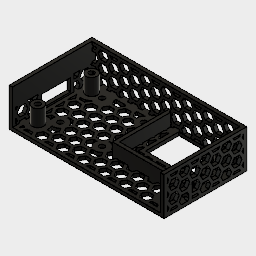
Enclosure Bottom (Autodesk Fusion 360 design; units mm, degrees)
Autodesk Fusion 360 part; units mm, degrees
(part 1 of 2)
sketch "Base and Side Wall" plane through (0, 0, 0) normal (0, 1, 0) x (1, 0, 0)
  line L0 (0, 0) -> (88.9, 0)
  line L1 (88.9, 0) -> (88.9, -47.6)
  line L2 (88.9, -47.6) -> (0, -47.6)
  line L3 (0, -47.6) -> (0, 0)
  line L4 (0, 0) -> (0, -2)
  line L5 (2, -2) -> (86.9, -2)
  line L6 (86.9, -2) -> (86.9, -47.6)
  line L7 (2, -47.6) -> (2, -2)
  dimension "d1" = 88.9
  dimension "d2" = 47.6
  dimension "d3" = 2
  dimension "d100" = 2
  measures "d1" distance of L0.start L0.end
  measures "d2" distance of L0.start L2.end
  measures "d3" distance of L0.start L4.end
extrude "Extrude1" add sketch "Base and Side Wall" along normal blind 2 contours L2 L5 L6 L7 makes body 1
extrude "Extrude2" add sketch "Base and Side Wall" along normal blind 22 separate body contours L0 L1 L2 L3 L4 L5 L6 L7 makes body 2
sketch "Board Construction Lines" plane through (0, 0, 0) normal (0, 1, 0) x (1, 0, 0)
  line L0 (4.75, -3.4956) -> (85.4, -3.5) construction
  line L1 (85.4, -3.5) -> (85.3525, -46.1425) construction
  line L2 (85.3525, -46.1425) -> (4.7511, -46.1014) construction
  line L3 (4.7511, -46.1014) -> (4.75, -3.4956) construction
  line L4 (4.75, -3.4956) -> (7.15, -3.5001) construction
  line L5 (7.15, -3.5001) -> (7.1569, -7.3501) construction
  line L6 (7.1569, -7.3501) -> (4.7569, -7.3456) construction
  line L7 (4.7569, -7.3456) -> (4.75, -3.4956) construction
  line L8 (85.4, -3.5) -> (82.15, -3.5001) construction
  line L9 (82.15, -3.5001) -> (82.1501, -7.3501) construction
  line L10 (82.1501, -7.3501) -> (85.4001, -7.35) construction
  line L11 (85.4001, -7.35) -> (85.4, -3.5) construction
  line L12 (4.7511, -46.1014) -> (7.1511, -46.1012) construction
  line L13 (7.1511, -46.1012) -> (7.1569, -38.2512) construction
  line L14 (7.1569, -38.2512) -> (4.7569, -38.2514) construction
  line L15 (4.7569, -38.2514) -> (4.7511, -46.1014) construction
  line L16 (85.3525, -46.1425) -> (82.1027, -46.1011) construction
  line L17 (82.1027, -46.1011) -> (82.1501, -38.2512) construction
  line L18 (82.1501, -38.2512) -> (85.3999, -38.2926) construction
  line L19 (85.3999, -38.2926) -> (85.3525, -46.1425) construction
  line L20 (7.1569, -7.3501) -> (82.1501, -7.3501) construction
  line L21 (82.1501, -7.3501) -> (82.1501, -38.2512) construction
  line L22 (82.1501, -38.2512) -> (7.1569, -38.2512) construction
  line L23 (7.1569, -38.2512) -> (7.1569, -7.3501) construction
  dimension "d18" = 80.65
  dimension "d20" = 2.4
  dimension "d21" = 3.25
  dimension "d22" = 3.85
  dimension "d23" = 7.85
  measures "d18" distance of L0.start L0.end
  measures "d20" distance of L0.start L4.end
  measures "d21" distance of L0.end L8.end
  measures "d22" distance of L0.end L10.end
  measures "d23" distance of L2.end L14.end
sketch "Standoffs" plane through (0, 2, 0) normal (0, 1, 0) x (-1, 0, 0)
  line L0 (-2, 47.6) -> (-86.9, 47.6)
  line L1 (-86.9, 47.6) -> (-86.9, 2)
  line L2 (-86.9, 2) -> (-2, 2)
  line L3 (-2, 2) -> (-2, 47.6)
  circle A0 centre (-7.1569, 7.3501) radius 1.5
  circle A1 centre (-7.147, 7.3545) radius 3.25
  circle A2 centre (-7.147, 7.3545) radius 1.5
  circle A3 centre (-82.1501, 7.3501) radius 1.5
  circle A4 centre (-82.1501, 7.3501) radius 3.25
  circle A5 centre (-82.1501, 38.2512) radius 1.5
  circle A6 centre (-82.1501, 38.2512) radius 3.25
  circle A7 centre (-7.1569, 38.2512) radius 1.5
  circle A8 centre (-7.1569, 38.2512) radius 3.25
  point P0 (-7.1569, 7.3501)
  point P1 (-82.1501, 7.3501)
  point P2 (-82.1501, 38.2512)
  point P3 (-7.1569, 38.2512)
  dimension "d29" = 3
  dimension "d31" = 3
  dimension "d32" = 6.5
  dimension "d33" = 3
  dimension "d34" = 6.5
  dimension "d37" = 3
  dimension "d38" = 6.5
  dimension "d41" = 3
  dimension "d42" = 6.5
  measures "d29" diameter of A0
  measures "d31" diameter of A2
  measures "d32" diameter of A1
  measures "d33" diameter of A3
  measures "d34" diameter of A4
  measures "d37" diameter of A5
  measures "d38" diameter of A6
  measures "d41" diameter of A7
  measures "d42" diameter of A8
extrude "Extrude3" add sketch "Standoffs" along normal blind 9.5 contours A1 | A4 | A6 bodies 1
sketch "Nut Holes" plane through (0, 0, 0) normal (0, 1, 0) x (1, 0, 0)
  line L0 (9.4069, -38.2546) -> (8.2848, -36.3043)
  line L1 (8.2848, -36.3043) -> (6.0348, -36.301)
  line L2 (6.0348, -36.301) -> (4.9069, -38.2478)
  line L3 (4.9069, -38.2478) -> (6.029, -40.1981)
  line L4 (6.029, -40.1981) -> (8.279, -40.2014)
  line L5 (8.279, -40.2014) -> (9.4069, -38.2546)
  line L6 (79.9001, -38.2512) -> (81.0251, -40.1998)
  line L7 (81.0251, -40.1998) -> (83.2751, -40.1998)
  line L8 (83.2751, -40.1998) -> (84.4001, -38.2512)
  line L9 (84.4001, -38.2512) -> (83.2751, -36.3026)
  line L10 (83.2751, -36.3026) -> (81.0251, -36.3026)
  line L11 (81.0251, -36.3026) -> (79.9001, -38.2512)
  line L12 (79.9001, -7.3501) -> (81.0251, -9.2987)
  line L13 (81.0251, -9.2987) -> (83.2751, -9.2987)
  line L14 (83.2751, -9.2987) -> (84.4001, -7.3501)
  line L15 (84.4001, -7.3501) -> (83.2751, -5.4016)
  line L16 (83.2751, -5.4016) -> (81.0251, -5.4016)
  line L17 (81.0251, -5.4016) -> (79.9001, -7.3501)
  line L18 (9.397, -7.3528) -> (8.2705, -5.4051)
  line L19 (8.2705, -5.4051) -> (6.0205, -5.4069)
  line L20 (6.0205, -5.4069) -> (4.897, -7.3563)
  line L21 (4.897, -7.3563) -> (6.0236, -9.304)
  line L22 (6.0236, -9.304) -> (8.2736, -9.3022)
  line L23 (8.2736, -9.3022) -> (9.397, -7.3528)
  point P0 (7.1569, -38.2512)
  point P1 (82.1501, -38.2512)
  point P2 (82.1501, -7.3501)
  point P3 (7.147, -7.3545)
  dimension "d205" = 4.5
  dimension "d206" = 4.5
  dimension "d207" = 4.5
  dimension "d208" = 4.5
  measures "d205" distance of L0.start L2.end
  measures "d206" distance of L6.start L8.end
  measures "d207" distance of L18.start L20.end
  measures "d208" distance of L12.start L14.end
extrude "Extrude4" add sketch "Standoffs" along normal blind 9.5 contours A8 bodies 1
extrude "Extrude5" cut sketch "Nut Holes" along normal blind 6 bodies 1
sketch "USB Port" plane through (0, 0, 0) normal (1, 0, 0) x (0, 0, -1)
  line L0 (-30.93, 3) -> (-14.33, 3)
  line L1 (-14.33, 3) -> (-14.33, 10)
  line L2 (-14.33, 10) -> (-30.93, 10)
  line L3 (-30.93, 10) -> (-30.93, 3)
  point P0 (-20.63, 6.5)
  point P1 (-20.63, 6.5)
  dimension "d49" = 16.6
  dimension "d50" = 7
  measures "d49" distance of L1.end L2.end
  measures "d50" distance of L0.end L1.end
extrude "Extrude6" cut sketch "USB Port" along normal blind 2 bodies 2
sketch "Bottom Honeycomb" plane through (0, 0, 0) normal (0, 1, 0) x (1, 0, 0)
  line L0 (77.1501, -5.9981) -> (12.1569, -5.9981) construction
  line L1 (12.1569, -5.9981) -> (12.1569, -45.6006) construction
  line L2 (12.1569, -45.6006) -> (77.1501, -45.6006) construction
  line L3 (77.1501, -45.6006) -> (77.1501, -5.9981) construction
  line L4 (47.6535, -25.7993) -> (46.1535, -23.2013)
  line L5 (46.1535, -23.2013) -> (43.1535, -23.2013)
  line L6 (43.1535, -23.2013) -> (41.6535, -25.7993)
  line L7 (41.6535, -25.7993) -> (43.1535, -28.3974)
  line L8 (43.1535, -28.3974) -> (46.1535, -28.3974)
  line L9 (46.1535, -28.3974) -> (47.6535, -25.7993)
  line L10 (41.6535, -29.2993) -> (40.1535, -26.7013)
  line L11 (40.1535, -26.7013) -> (37.1535, -26.7013)
  line L12 (37.1535, -26.7013) -> (35.6535, -29.2993)
  line L13 (35.6535, -29.2993) -> (37.1535, -31.8974)
  line L14 (37.1535, -31.8974) -> (40.1535, -31.8974)
  line L15 (40.1535, -31.8974) -> (41.6535, -29.2993)
  line L16 (35.6535, -25.7993) -> (34.1535, -23.2013)
  line L17 (34.1535, -23.2013) -> (31.1535, -23.2013)
  line L18 (31.1535, -23.2013) -> (29.6535, -25.7993)
  line L19 (29.6535, -25.7993) -> (31.1535, -28.3974)
  line L20 (31.1535, -28.3974) -> (34.1535, -28.3974)
  line L21 (34.1535, -28.3974) -> (35.6535, -25.7993)
  line L22 (22.1535, -23.2013) -> (19.1535, -23.2013)
  line L23 (19.1535, -23.2013) -> (17.6535, -25.7993)
  line L24 (17.6535, -25.7993) -> (19.1535, -28.3974)
  line L25 (19.1535, -28.3974) -> (22.1535, -28.3974)
  line L26 (22.1535, -28.3974) -> (23.6535, -25.7993)
  line L27 (23.6535, -25.7993) -> (22.1535, -23.2013)
  line L28 (11.6535, -25.7993) -> (10.1535, -23.2013)
  line L29 (10.1535, -23.2013) -> (7.1535, -23.2013)
  line L30 (7.1535, -23.2013) -> (5.6535, -25.7993)
  line L31 (5.6535, -25.7993) -> (7.1535, -28.3974)
  line L32 (7.1535, -28.3974) -> (10.1535, -28.3974)
  line L33 (10.1535, -28.3974) -> (11.6535, -25.7993)
  line L34 (59.6535, -25.7993) -> (58.1535, -23.2013)
  line L35 (58.1535, -23.2013) -> (55.1535, -23.2013)
  line L36 (55.1535, -23.2013) -> (53.6535, -25.7993)
  line L37 (53.6535, -25.7993) -> (55.1535, -28.3974)
  line L38 (55.1535, -28.3974) -> (58.1535, -28.3974)
  line L39 (58.1535, -28.3974) -> (59.6535, -25.7993)
  line L40 (71.6535, -25.7993) -> (70.1535, -23.2013)
  line L41 (70.1535, -23.2013) -> (67.1535, -23.2013)
  line L42 (67.1535, -23.2013) -> (65.6535, -25.7993)
  line L43 (65.6535, -25.7993) -> (67.1535, -28.3974)
  line L44 (67.1535, -28.3974) -> (70.1535, -28.3974)
  line L45 (70.1535, -28.3974) -> (71.6535, -25.7993)
  line L46 (83.6535, -25.7993) -> (82.1535, -23.2013)
  line L47 (82.1535, -23.2013) -> (79.1535, -23.2013)
  line L48 (79.1535, -23.2013) -> (77.6535, -25.7993)
  line L49 (77.6535, -25.7993) -> (79.1535, -28.3974)
  line L50 (79.1535, -28.3974) -> (82.1535, -28.3974)
  line L51 (82.1535, -28.3974) -> (83.6535, -25.7993)
  line L52 (29.6535, -29.2993) -> (28.1535, -26.7013)
  line L53 (28.1535, -26.7013) -> (25.1535, -26.7013)
  line L54 (25.1535, -26.7013) -> (23.6535, -29.2993)
  line L55 (23.6535, -29.2993) -> (25.1535, -31.8974)
  line L56 (25.1535, -31.8974) -> (28.1535, -31.8974)
  line L57 (28.1535, -31.8974) -> (29.6535, -29.2993)
  line L58 (16.1535, -26.7013) -> (13.1535, -26.7013)
  line L59 (13.1535, -26.7013) -> (11.6535, -29.2993)
  line L60 (11.6535, -29.2993) -> (13.1535, -31.8974)
  line L61 (13.1535, -31.8974) -> (16.1535, -31.8974)
  line L62 (16.1535, -31.8974) -> (17.6535, -29.2993)
  line L63 (17.6535, -29.2993) -> (16.1535, -26.7013)
  line L64 (53.6535, -29.2993) -> (52.1535, -26.7013)
  line L65 (52.1535, -26.7013) -> (49.1535, -26.7013)
  line L66 (49.1535, -26.7013) -> (47.6535, -29.2993)
  line L67 (47.6535, -29.2993) -> (49.1535, -31.8974)
  line L68 (49.1535, -31.8974) -> (52.1535, -31.8974)
  line L69 (52.1535, -31.8974) -> (53.6535, -29.2993)
  line L70 (65.6535, -29.2993) -> (64.1535, -26.7013)
  line L71 (64.1535, -26.7013) -> (61.1535, -26.7013)
  line L72 (61.1535, -26.7013) -> (59.6535, -29.2993)
  line L73 (59.6535, -29.2993) -> (61.1535, -31.8974)
  line L74 (61.1535, -31.8974) -> (64.1535, -31.8974)
  line L75 (64.1535, -31.8974) -> (65.6535, -29.2993)
  line L76 (76.1535, -26.7013) -> (73.1535, -26.7013)
  line L77 (73.1535, -26.7013) -> (71.6535, -29.2993)
  line L78 (71.6535, -29.2993) -> (73.1535, -31.8974)
  line L79 (73.1535, -31.8974) -> (76.1535, -31.8974)
  line L80 (76.1535, -31.8974) -> (77.6535, -29.2993)
  line L81 (77.6535, -29.2993) -> (76.1535, -26.7013)
  line L82 (17.6535, -22.2993) -> (16.1535, -19.7013)
  line L83 (16.1535, -19.7013) -> (13.1535, -19.7013)
  line L84 (13.1535, -19.7013) -> (11.6535, -22.2993)
  line L85 (11.6535, -22.2993) -> (13.1535, -24.8974)
  line L86 (13.1535, -24.8974) -> (16.1535, -24.8974)
  line L87 (16.1535, -24.8974) -> (17.6535, -22.2993)
  line L88 (29.6535, -22.2993) -> (28.1535, -19.7013)
  line L89 (28.1535, -19.7013) -> (25.1535, -19.7013)
  line L90 (25.1535, -19.7013) -> (23.6535, -22.2993)
  line L91 (23.6535, -22.2993) -> (25.1535, -24.8974)
  line L92 (28.1535, -24.8974) -> (29.6535, -22.2993)
  line L93 (25.1535, -24.8974) -> (28.1535, -24.8974)
  line L94 (41.6535, -22.2993) -> (40.1535, -19.7013)
  line L95 (40.1535, -19.7013) -> (37.1535, -19.7013)
  line L96 (37.1535, -19.7013) -> (35.6535, -22.2993)
  line L97 (35.6535, -22.2993) -> (37.1535, -24.8974)
  line L98 (40.1535, -24.8974) -> (41.6535, -22.2993)
  line L99 (37.1535, -24.8974) -> (40.1535, -24.8974)
  line L100 (53.6535, -22.2993) -> (52.1535, -19.7013)
  line L101 (52.1535, -19.7013) -> (49.1535, -19.7013)
  line L102 (49.1535, -19.7013) -> (47.6535, -22.2993)
  line L103 (47.6535, -22.2993) -> (49.1535, -24.8974)
  line L104 (52.1535, -24.8974) -> (53.6535, -22.2993)
  line L105 (49.1535, -24.8974) -> (52.1535, -24.8974)
  line L106 (65.6535, -22.2993) -> (64.1535, -19.7013)
  line L107 (64.1535, -19.7013) -> (61.1535, -19.7013)
  line L108 (61.1535, -19.7013) -> (59.6535, -22.2993)
  line L109 (59.6535, -22.2993) -> (61.1535, -24.8974)
  line L110 (64.1535, -24.8974) -> (65.6535, -22.2993)
  line L111 (61.1535, -24.8974) -> (64.1535, -24.8974)
  line L112 (77.6535, -22.2993) -> (76.1535, -19.7013)
  line L113 (76.1535, -19.7013) -> (73.1535, -19.7013)
  line L114 (73.1535, -19.7013) -> (71.6535, -22.2993)
  line L115 (71.6535, -22.2993) -> (73.1535, -24.8974)
  line L116 (76.1535, -24.8974) -> (77.6535, -22.2993)
  line L117 (73.1535, -24.8974) -> (76.1535, -24.8974)
  line L118 (11.6535, -18.7993) -> (10.1535, -16.2013)
  line L119 (10.1535, -16.2013) -> (7.1535, -16.2013)
  line L120 (7.1535, -16.2013) -> (5.6535, -18.7993)
  line L121 (5.6535, -18.7993) -> (7.1535, -21.3974)
  line L122 (7.1535, -21.3974) -> (10.1535, -21.3974)
  line L123 (10.1535, -21.3974) -> (11.6535, -18.7993)
  line L124 (23.6535, -18.7993) -> (22.1535, -16.2013)
  line L125 (22.1535, -16.2013) -> (19.1535, -16.2013)
  line L126 (19.1535, -16.2013) -> (17.6535, -18.7993)
  line L127 (17.6535, -18.7993) -> (19.1535, -21.3974)
  line L128 (22.1535, -21.3974) -> (23.6535, -18.7993)
  line L129 (19.1535, -21.3974) -> (22.1535, -21.3974)
  line L130 (35.6535, -18.7993) -> (34.1535, -16.2013)
  line L131 (34.1535, -16.2013) -> (31.1535, -16.2013)
  line L132 (31.1535, -16.2013) -> (29.6535, -18.7993)
  line L133 (29.6535, -18.7993) -> (31.1535, -21.3974)
  line L134 (34.1535, -21.3974) -> (35.6535, -18.7993)
  line L135 (31.1535, -21.3974) -> (34.1535, -21.3974)
  line L136 (47.6535, -18.7993) -> (46.1535, -16.2013)
  line L137 (46.1535, -16.2013) -> (43.1535, -16.2013)
  line L138 (43.1535, -16.2013) -> (41.6535, -18.7993)
  line L139 (41.6535, -18.7993) -> (43.1535, -21.3974)
  line L140 (46.1535, -21.3974) -> (47.6535, -18.7993)
  line L141 (43.1535, -21.3974) -> (46.1535, -21.3974)
  line L142 (59.6535, -18.7993) -> (58.1535, -16.2013)
  line L143 (58.1535, -16.2013) -> (55.1535, -16.2013)
  line L144 (55.1535, -16.2013) -> (53.6535, -18.7993)
  line L145 (53.6535, -18.7993) -> (55.1535, -21.3974)
  line L146 (58.1535, -21.3974) -> (59.6535, -18.7993)
  line L147 (55.1535, -21.3974) -> (58.1535, -21.3974)
  line L148 (71.6535, -18.7993) -> (70.1535, -16.2013)
  line L149 (70.1535, -16.2013) -> (67.1535, -16.2013)
  line L150 (67.1535, -16.2013) -> (65.6535, -18.7993)
  line L151 (65.6535, -18.7993) -> (67.1535, -21.3974)
  line L152 (70.1535, -21.3974) -> (71.6535, -18.7993)
  line L153 (67.1535, -21.3974) -> (70.1535, -21.3974)
  line L154 (83.6535, -18.7993) -> (82.1535, -16.2013)
  line L155 (82.1535, -16.2013) -> (79.1535, -16.2013)
  line L156 (79.1535, -16.2013) -> (77.6535, -18.7993)
  line L157 (77.6535, -18.7993) -> (79.1535, -21.3974)
  line L158 (82.1535, -21.3974) -> (83.6535, -18.7993)
  line L159 (79.1535, -21.3974) -> (82.1535, -21.3974)
  line L160 (23.6535, -11.7993) -> (22.1535, -9.2013)
  line L161 (22.1535, -9.2013) -> (19.1535, -9.2013)
  line L162 (19.1535, -9.2013) -> (17.6535, -11.7993)
  line L163 (17.6535, -11.7993) -> (19.1535, -14.3974)
  line L164 (22.1535, -14.3974) -> (23.6535, -11.7993)
  line L165 (19.1535, -14.3974) -> (22.1535, -14.3974)
  line L166 (35.6535, -11.7993) -> (34.1535, -9.2013)
  line L167 (34.1535, -9.2013) -> (31.1535, -9.2013)
  line L168 (31.1535, -9.2013) -> (29.6535, -11.7993)
  line L169 (29.6535, -11.7993) -> (31.1535, -14.3974)
  line L170 (34.1535, -14.3974) -> (35.6535, -11.7993)
  line L171 (31.1535, -14.3974) -> (34.1535, -14.3974)
  line L172 (47.6535, -11.7993) -> (46.1535, -9.2013)
  line L173 (46.1535, -9.2013) -> (43.1535, -9.2013)
  line L174 (43.1535, -9.2013) -> (41.6535, -11.7993)
  line L175 (41.6535, -11.7993) -> (43.1535, -14.3974)
  line L176 (46.1535, -14.3974) -> (47.6535, -11.7993)
  line L177 (43.1535, -14.3974) -> (46.1535, -14.3974)
  line L178 (59.6535, -11.7993) -> (58.1535, -9.2013)
  line L179 (58.1535, -9.2013) -> (55.1535, -9.2013)
  line L180 (55.1535, -9.2013) -> (53.6535, -11.7993)
  line L181 (53.6535, -11.7993) -> (55.1535, -14.3974)
  line L182 (58.1535, -14.3974) -> (59.6535, -11.7993)
  line L183 (55.1535, -14.3974) -> (58.1535, -14.3974)
  line L184 (71.6535, -11.7993) -> (70.1535, -9.2013)
  line L185 (70.1535, -9.2013) -> (67.1535, -9.2013)
  line L186 (67.1535, -9.2013) -> (65.6535, -11.7993)
  line L187 (65.6535, -11.7993) -> (67.1535, -14.3974)
  line L188 (70.1535, -14.3974) -> (71.6535, -11.7993)
  line L189 (67.1535, -14.3974) -> (70.1535, -14.3974)
  line L190 (17.6535, -15.2993) -> (16.1535, -12.7013)
  line L191 (16.1535, -12.7013) -> (13.1535, -12.7013)
  line L192 (13.1535, -12.7013) -> (11.6535, -15.2993)
  line L193 (11.6535, -15.2993) -> (13.1535, -17.8974)
  line L194 (13.1535, -17.8974) -> (16.1535, -17.8974)
  line L195 (16.1535, -17.8974) -> (17.6535, -15.2993)
  line L196 (29.6535, -15.2993) -> (28.1535, -12.7013)
  line L197 (28.1535, -12.7013) -> (25.1535, -12.7013)
  line L198 (25.1535, -12.7013) -> (23.6535, -15.2993)
  line L199 (23.6535, -15.2993) -> (25.1535, -17.8974)
  line L200 (28.1535, -17.8974) -> (29.6535, -15.2993)
  line L201 (25.1535, -17.8974) -> (28.1535, -17.8974)
  line L202 (41.6535, -15.2993) -> (40.1535, -12.7013)
  line L203 (40.1535, -12.7013) -> (37.1535, -12.7013)
  line L204 (37.1535, -12.7013) -> (35.6535, -15.2993)
  line L205 (35.6535, -15.2993) -> (37.1535, -17.8974)
  line L206 (40.1535, -17.8974) -> (41.6535, -15.2993)
  line L207 (37.1535, -17.8974) -> (40.1535, -17.8974)
  line L208 (53.6535, -15.2993) -> (52.1535, -12.7013)
  line L209 (52.1535, -12.7013) -> (49.1535, -12.7013)
  line L210 (49.1535, -12.7013) -> (47.6535, -15.2993)
  line L211 (47.6535, -15.2993) -> (49.1535, -17.8974)
  line L212 (52.1535, -17.8974) -> (53.6535, -15.2993)
  line L213 (49.1535, -17.8974) -> (52.1535, -17.8974)
  line L214 (65.6535, -15.2993) -> (64.1535, -12.7013)
  line L215 (64.1535, -12.7013) -> (61.1535, -12.7013)
  line L216 (61.1535, -12.7013) -> (59.6535, -15.2993)
  line L217 (59.6535, -15.2993) -> (61.1535, -17.8974)
  line L218 (64.1535, -17.8974) -> (65.6535, -15.2993)
  line L219 (61.1535, -17.8974) -> (64.1535, -17.8974)
  line L220 (77.6535, -15.2993) -> (76.1535, -12.7013)
  line L221 (76.1535, -12.7013) -> (73.1535, -12.7013)
  line L222 (73.1535, -12.7013) -> (71.6535, -15.2993)
  line L223 (71.6535, -15.2993) -> (73.1535, -17.8974)
  line L224 (76.1535, -17.8974) -> (77.6535, -15.2993)
  line L225 (73.1535, -17.8974) -> (76.1535, -17.8974)
  line L226 (23.6535, -32.7993) -> (22.1535, -30.2013)
  line L227 (22.1535, -30.2013) -> (19.1535, -30.2013)
  line L228 (19.1535, -30.2013) -> (17.6535, -32.7993)
  line L229 (17.6535, -32.7993) -> (19.1535, -35.3974)
  line L230 (22.1535, -35.3974) -> (23.6535, -32.7993)
  line L231 (19.1535, -35.3974) -> (22.1535, -35.3974)
  line L232 (35.6535, -32.7993) -> (34.1535, -30.2013)
  line L233 (34.1535, -30.2013) -> (31.1535, -30.2013)
  line L234 (31.1535, -30.2013) -> (29.6535, -32.7993)
  line L235 (29.6535, -32.7993) -> (31.1535, -35.3974)
  line L236 (34.1535, -35.3974) -> (35.6535, -32.7993)
  line L237 (31.1535, -35.3974) -> (34.1535, -35.3974)
  line L238 (47.6535, -32.7993) -> (46.1535, -30.2013)
  line L239 (46.1535, -30.2013) -> (43.1535, -30.2013)
  line L240 (43.1535, -30.2013) -> (41.6535, -32.7993)
  line L241 (41.6535, -32.7993) -> (43.1535, -35.3974)
  line L242 (46.1535, -35.3974) -> (47.6535, -32.7993)
  line L243 (43.1535, -35.3974) -> (46.1535, -35.3974)
  line L244 (59.6535, -32.7993) -> (58.1535, -30.2013)
  line L245 (58.1535, -30.2013) -> (55.1535, -30.2013)
  line L246 (55.1535, -30.2013) -> (53.6535, -32.7993)
  line L247 (53.6535, -32.7993) -> (55.1535, -35.3974)
  line L248 (58.1535, -35.3974) -> (59.6535, -32.7993)
  line L249 (55.1535, -35.3974) -> (58.1535, -35.3974)
  line L250 (71.6535, -32.7993) -> (70.1535, -30.2013)
  line L251 (70.1535, -30.2013) -> (67.1535, -30.2013)
  line L252 (67.1535, -30.2013) -> (65.6535, -32.7993)
  line L253 (65.6535, -32.7993) -> (67.1535, -35.3974)
  line L254 (70.1535, -35.3974) -> (71.6535, -32.7993)
  line L255 (67.1535, -35.3974) -> (70.1535, -35.3974)
  line L256 (17.6535, -36.2993) -> (16.1535, -33.7013)
  line L257 (16.1535, -33.7013) -> (13.1535, -33.7013)
  line L258 (13.1535, -33.7013) -> (11.6535, -36.2993)
  line L259 (11.6535, -36.2993) -> (13.1535, -38.8974)
  line L260 (13.1535, -38.8974) -> (16.1535, -38.8974)
  line L261 (16.1535, -38.8974) -> (17.6535, -36.2993)
  line L262 (29.6535, -36.2993) -> (28.1535, -33.7013)
  line L263 (28.1535, -33.7013) -> (25.1535, -33.7013)
  line L264 (25.1535, -33.7013) -> (23.6535, -36.2993)
  line L265 (23.6535, -36.2993) -> (25.1535, -38.8974)
  line L266 (28.1535, -38.8974) -> (29.6535, -36.2993)
  line L267 (25.1535, -38.8974) -> (28.1535, -38.8974)
  line L268 (41.6535, -36.2993) -> (40.1535, -33.7013)
  line L269 (40.1535, -33.7013) -> (37.1535, -33.7013)
  line L270 (37.1535, -33.7013) -> (35.6535, -36.2993)
  line L271 (35.6535, -36.2993) -> (37.1535, -38.8974)
  line L272 (40.1535, -38.8974) -> (41.6535, -36.2993)
  line L273 (37.1535, -38.8974) -> (40.1535, -38.8974)
  line L274 (53.6535, -36.2993) -> (52.1535, -33.7013)
  line L275 (52.1535, -33.7013) -> (49.1535, -33.7013)
  line L276 (49.1535, -33.7013) -> (47.6535, -36.2993)
  line L277 (47.6535, -36.2993) -> (49.1535, -38.8974)
  line L278 (52.1535, -38.8974) -> (53.6535, -36.2993)
  line L279 (49.1535, -38.8974) -> (52.1535, -38.8974)
  line L280 (65.6535, -36.2993) -> (64.1535, -33.7013)
  line L281 (64.1535, -33.7013) -> (61.1535, -33.7013)
  line L282 (61.1535, -33.7013) -> (59.6535, -36.2993)
  line L283 (59.6535, -36.2993) -> (61.1535, -38.8974)
  line L284 (64.1535, -38.8974) -> (65.6535, -36.2993)
  line L285 (61.1535, -38.8974) -> (64.1535, -38.8974)
  line L286 (77.6535, -36.2993) -> (76.1535, -33.7013)
  line L287 (76.1535, -33.7013) -> (73.1535, -33.7013)
  line L288 (73.1535, -33.7013) -> (71.6535, -36.2993)
  line L289 (71.6535, -36.2993) -> (73.1535, -38.8974)
  line L290 (76.1535, -38.8974) -> (77.6535, -36.2993)
  line L291 (73.1535, -38.8974) -> (76.1535, -38.8974)
  line L292 (23.6535, -39.7993) -> (22.1535, -37.2013)
  line L293 (22.1535, -37.2013) -> (19.1535, -37.2013)
  line L294 (19.1535, -37.2013) -> (17.6535, -39.7993)
  line L295 (17.6535, -39.7993) -> (19.1535, -42.3974)
  line L296 (22.1535, -42.3974) -> (23.6535, -39.7993)
  line L297 (19.1535, -42.3974) -> (22.1535, -42.3974)
  line L298 (35.6535, -39.7993) -> (34.1535, -37.2013)
  line L299 (34.1535, -37.2013) -> (31.1535, -37.2013)
  line L300 (31.1535, -37.2013) -> (29.6535, -39.7993)
  line L301 (29.6535, -39.7993) -> (31.1535, -42.3974)
  line L302 (34.1535, -42.3974) -> (35.6535, -39.7993)
  line L303 (31.1535, -42.3974) -> (34.1535, -42.3974)
  line L304 (47.6535, -39.7993) -> (46.1535, -37.2013)
  line L305 (46.1535, -37.2013) -> (43.1535, -37.2013)
  line L306 (43.1535, -37.2013) -> (41.6535, -39.7993)
  line L307 (41.6535, -39.7993) -> (43.1535, -42.3974)
  line L308 (46.1535, -42.3974) -> (47.6535, -39.7993)
  line L309 (43.1535, -42.3974) -> (46.1535, -42.3974)
  line L310 (59.6535, -39.7993) -> (58.1535, -37.2013)
  line L311 (58.1535, -37.2013) -> (55.1535, -37.2013)
  line L312 (55.1535, -37.2013) -> (53.6535, -39.7993)
  line L313 (53.6535, -39.7993) -> (55.1535, -42.3974)
  line L314 (58.1535, -42.3974) -> (59.6535, -39.7993)
  line L315 (55.1535, -42.3974) -> (58.1535, -42.3974)
  line L316 (71.6535, -39.7993) -> (70.1535, -37.2013)
  line L317 (70.1535, -37.2013) -> (67.1535, -37.2013)
  line L318 (67.1535, -37.2013) -> (65.6535, -39.7993)
  line L319 (65.6535, -39.7993) -> (67.1535, -42.3974)
  line L320 (70.1535, -42.3974) -> (71.6535, -39.7993)
  line L321 (67.1535, -42.3974) -> (70.1535, -42.3974)
  line L322 (17.6535, -8.2993) -> (16.1535, -5.7013)
  line L323 (16.1535, -5.7013) -> (13.1535, -5.7013)
  line L324 (13.1535, -5.7013) -> (11.6535, -8.2993)
  line L325 (11.6535, -8.2993) -> (13.1535, -10.8974)
  line L326 (13.1535, -10.8974) -> (16.1535, -10.8974)
  line L327 (16.1535, -10.8974) -> (17.6535, -8.2993)
  line L328 (29.6535, -8.2993) -> (28.1535, -5.7013)
  line L329 (28.1535, -5.7013) -> (25.1535, -5.7013)
  line L330 (25.1535, -5.7013) -> (23.6535, -8.2993)
  line L331 (23.6535, -8.2993) -> (25.1535, -10.8974)
  line L332 (28.1535, -10.8974) -> (29.6535, -8.2993)
  line L333 (25.1535, -10.8974) -> (28.1535, -10.8974)
  line L334 (41.6535, -8.2993) -> (40.1535, -5.7013)
  line L335 (40.1535, -5.7013) -> (37.1535, -5.7013)
  line L336 (37.1535, -5.7013) -> (35.6535, -8.2993)
  line L337 (35.6535, -8.2993) -> (37.1535, -10.8974)
  line L338 (40.1535, -10.8974) -> (41.6535, -8.2993)
  line L339 (37.1535, -10.8974) -> (40.1535, -10.8974)
  line L340 (53.6535, -8.2993) -> (52.1535, -5.7013)
  line L341 (52.1535, -5.7013) -> (49.1535, -5.7013)
  line L342 (49.1535, -5.7013) -> (47.6535, -8.2993)
  line L343 (47.6535, -8.2993) -> (49.1535, -10.8974)
  line L344 (52.1535, -10.8974) -> (53.6535, -8.2993)
  line L345 (49.1535, -10.8974) -> (52.1535, -10.8974)
  line L346 (65.6535, -8.2993) -> (64.1535, -5.7013)
  line L347 (64.1535, -5.7013) -> (61.1535, -5.7013)
  line L348 (61.1535, -5.7013) -> (59.6535, -8.2993)
  line L349 (59.6535, -8.2993) -> (61.1535, -10.8974)
  line L350 (64.1535, -10.8974) -> (65.6535, -8.2993)
  line L351 (61.1535, -10.8974) -> (64.1535, -10.8974)
  line L352 (77.6535, -8.2993) -> (76.1535, -5.7013)
  line L353 (76.1535, -5.7013) -> (73.1535, -5.7013)
  line L354 (73.1535, -5.7013) -> (71.6535, -8.2993)
  line L355 (71.6535, -8.2993) -> (73.1535, -10.8974)
  line L356 (76.1535, -10.8974) -> (77.6535, -8.2993)
  line L357 (73.1535, -10.8974) -> (76.1535, -10.8974)
  line L358 (35.6535, -8.2993) -> (41.6535, -8.2993) construction
  line L359 (38.6535, -5.7013) -> (38.6535, -10.8974) construction
  line L360 (47.6535, -8.2993) -> (53.6535, -8.2993) construction
  line L361 (50.6535, -5.7013) -> (50.6535, -10.8974) construction
  line L362 (17.6535, -4.7993) -> (19.1535, -7.3974)
  line L363 (19.1535, -7.3974) -> (22.1535, -7.3974)
  line L364 (22.1535, -7.3974) -> (23.6535, -4.7993)
  line L365 (23.6535, -4.7993) -> (22.1535, -2.2013)
  line L366 (22.1535, -2.2013) -> (19.1535, -2.2013)
  line L367 (19.1535, -2.2013) -> (17.6535, -4.7993)
  line L368 (29.6535, -4.7993) -> (31.1535, -7.3974)
  line L369 (31.1535, -7.3974) -> (34.1535, -7.3974)
  line L370 (34.1535, -7.3974) -> (35.6535, -4.7993)
  line L371 (35.6535, -4.7993) -> (34.1535, -2.2013)
  line L372 (31.1535, -2.2013) -> (29.6535, -4.7993)
  line L373 (34.1535, -2.2013) -> (31.1535, -2.2013)
  line L374 (41.6535, -4.7993) -> (43.1535, -7.3974)
  line L375 (43.1535, -7.3974) -> (46.1535, -7.3974)
  line L376 (46.1535, -7.3974) -> (47.6535, -4.7993)
  line L377 (47.6535, -4.7993) -> (46.1535, -2.2013)
  line L378 (43.1535, -2.2013) -> (41.6535, -4.7993)
  line L379 (46.1535, -2.2013) -> (43.1535, -2.2013)
  line L380 (53.6535, -4.7993) -> (55.1535, -7.3974)
  line L381 (55.1535, -7.3974) -> (58.1535, -7.3974)
  line L382 (58.1535, -7.3974) -> (59.6535, -4.7993)
  line L383 (59.6535, -4.7993) -> (58.1535, -2.2013)
  line L384 (55.1535, -2.2013) -> (53.6535, -4.7993)
  line L385 (58.1535, -2.2013) -> (55.1535, -2.2013)
  line L386 (65.6535, -4.7993) -> (67.1535, -7.3974)
  line L387 (67.1535, -7.3974) -> (70.1535, -7.3974)
  line L388 (70.1535, -7.3974) -> (71.6535, -4.7993)
  line L389 (71.6535, -4.7993) -> (70.1535, -2.2013)
  line L390 (67.1535, -2.2013) -> (65.6535, -4.7993)
  line L391 (70.1535, -2.2013) -> (67.1535, -2.2013)
  line L392 (29.6535, -43.2993) -> (28.1535, -40.7013)
  line L393 (28.1535, -40.7013) -> (25.1535, -40.7013)
  line L394 (25.1535, -40.7013) -> (23.6535, -43.2993)
  line L395 (23.6535, -43.2993) -> (25.1535, -45.8974)
  line L396 (28.1535, -45.8974) -> (29.6535, -43.2993)
  line L397 (25.1535, -45.8974) -> (28.1535, -45.8974)
  line L398 (41.6535, -43.2993) -> (40.1535, -40.7013)
  line L399 (40.1535, -40.7013) -> (37.1535, -40.7013)
  line L400 (37.1535, -40.7013) -> (35.6535, -43.2993)
  line L401 (35.6535, -43.2993) -> (37.1535, -45.8974)
  line L402 (40.1535, -45.8974) -> (41.6535, -43.2993)
  line L403 (37.1535, -45.8974) -> (40.1535, -45.8974)
  line L404 (53.6535, -43.2993) -> (52.1535, -40.7013)
  line L405 (52.1535, -40.7013) -> (49.1535, -40.7013)
  line L406 (49.1535, -40.7013) -> (47.6535, -43.2993)
  line L407 (47.6535, -43.2993) -> (49.1535, -45.8974)
  line L408 (52.1535, -45.8974) -> (53.6535, -43.2993)
  line L409 (49.1535, -45.8974) -> (52.1535, -45.8974)
  line L410 (65.6535, -43.2993) -> (64.1535, -40.7013)
  line L411 (64.1535, -40.7013) -> (61.1535, -40.7013)
  line L412 (61.1535, -40.7013) -> (59.6535, -43.2993)
  line L413 (59.6535, -43.2993) -> (61.1535, -45.8974)
  line L414 (64.1535, -45.8974) -> (65.6535, -43.2993)
  line L415 (61.1535, -45.8974) -> (64.1535, -45.8974)
  line L416 (77.6535, -43.2993) -> (76.1535, -40.7013)
  line L417 (76.1535, -40.7013) -> (73.1535, -40.7013)
  line L418 (73.1535, -40.7013) -> (71.6535, -43.2993)
  line L419 (71.6535, -43.2993) -> (73.1535, -45.8974)
  line L420 (76.1535, -45.8974) -> (77.6535, -43.2993)
  line L421 (73.1535, -45.8974) -> (76.1535, -45.8974)
  line L422 (17.6535, -43.2993) -> (16.1535, -40.7013)
  line L423 (16.1535, -40.7013) -> (13.1535, -40.7013)
  line L424 (13.1535, -40.7013) -> (11.6535, -43.2993)
  line L425 (11.6535, -43.2993) -> (13.1535, -45.8974)
  line L426 (13.1535, -45.8974) -> (16.1535, -45.8974)
  line L427 (16.1535, -45.8974) -> (17.6535, -43.2993)
  line L428 (5.6535, -11.7993) -> (7.1535, -14.3974)
  line L429 (7.1535, -14.3974) -> (10.1535, -14.3974)
  line L430 (10.1535, -14.3974) -> (11.6535, -11.7993)
  line L431 (11.6535, -11.7993) -> (10.1535, -9.2013)
  line L432 (10.1535, -9.2013) -> (7.1535, -9.2013)
  line L433 (7.1535, -9.2013) -> (5.6535, -11.7993)
  line L434 (5.6535, -32.7993) -> (7.1535, -35.3974)
  line L435 (7.1535, -35.3974) -> (10.1535, -35.3974)
  line L436 (10.1535, -35.3974) -> (11.6535, -32.7993)
  line L437 (11.6535, -32.7993) -> (10.1535, -30.2013)
  line L438 (7.1535, -30.2013) -> (5.6535, -32.7993)
  line L439 (10.1535, -30.2013) -> (7.1535, -30.2013)
  line L440 (83.6535, -11.7993) -> (82.1535, -9.2013)
  line L441 (82.1535, -9.2013) -> (79.1535, -9.2013)
  line L442 (79.1535, -9.2013) -> (77.6535, -11.7993)
  line L443 (77.6535, -11.7993) -> (79.1535, -14.3974)
  line L444 (79.1535, -14.3974) -> (82.1535, -14.3974)
  line L445 (82.1535, -14.3974) -> (83.6535, -11.7993)
  line L446 (77.6535, -32.7993) -> (79.1535, -35.3974)
  line L447 (79.1535, -35.3974) -> (82.1535, -35.3974)
  line L448 (82.1535, -35.3974) -> (83.6535, -32.7993)
  line L449 (83.6535, -32.7993) -> (82.1535, -30.2013)
  line L450 (79.1535, -30.2013) -> (77.6535, -32.7993)
  line L451 (82.1535, -30.2013) -> (79.1535, -30.2013)
  line L452 (71.6535, -46.7993) -> (70.1535, -44.2013)
  line L453 (70.1535, -44.2013) -> (67.1535, -44.2013)
  line L454 (67.1535, -44.2013) -> (65.6535, -46.7993)
  line L455 (65.6535, -46.7993) -> (67.1535, -49.3974)
  line L456 (67.1535, -49.3974) -> (70.1535, -49.3974)
  line L457 (70.1535, -49.3974) -> (71.6535, -46.7993)
  line L458 (59.6535, -46.7993) -> (58.1535, -44.2013)
  line L459 (58.1535, -44.2013) -> (55.1535, -44.2013)
  line L460 (55.1535, -44.2013) -> (53.6535, -46.7993)
  line L461 (53.6535, -46.7993) -> (55.1535, -49.3974)
  line L462 (58.1535, -49.3974) -> (59.6535, -46.7993)
  line L463 (55.1535, -49.3974) -> (58.1535, -49.3974)
  line L464 (47.6535, -46.7993) -> (46.1535, -44.2013)
  line L465 (46.1535, -44.2013) -> (43.1535, -44.2013)
  line L466 (43.1535, -44.2013) -> (41.6535, -46.7993)
  line L467 (41.6535, -46.7993) -> (43.1535, -49.3974)
  line L468 (46.1535, -49.3974) -> (47.6535, -46.7993)
  line L469 (43.1535, -49.3974) -> (46.1535, -49.3974)
  line L470 (35.6535, -46.7993) -> (34.1535, -44.2013)
  line L471 (34.1535, -44.2013) -> (31.1535, -44.2013)
  line L472 (31.1535, -44.2013) -> (29.6535, -46.7993)
  line L473 (29.6535, -46.7993) -> (31.1535, -49.3974)
  line L474 (34.1535, -49.3974) -> (35.6535, -46.7993)
  line L475 (31.1535, -49.3974) -> (34.1535, -49.3974)
  line L476 (23.6535, -46.7993) -> (22.1535, -44.2013)
  line L477 (22.1535, -44.2013) -> (19.1535, -44.2013)
  line L478 (19.1535, -44.2013) -> (17.6535, -46.7993)
  line L479 (17.6535, -46.7993) -> (19.1535, -49.3974)
  line L480 (22.1535, -49.3974) -> (23.6535, -46.7993)
  line L481 (19.1535, -49.3974) -> (22.1535, -49.3974)
  line L482 (5.6535, -46.7993) -> (7.1535, -49.3974)
  line L483 (7.1535, -49.3974) -> (10.1535, -49.3974)
  line L484 (10.1535, -49.3974) -> (11.6535, -46.7993)
  line L485 (11.6535, -46.7993) -> (10.1535, -44.2013)
  line L486 (10.1535, -44.2013) -> (7.1535, -44.2013)
  line L487 (7.1535, -44.2013) -> (5.6535, -46.7993)
  line L488 (2, -2) -> (86.9, -2)
  line L489 (86.9, -2) -> (2, -2)
  line L490 (4, -4) -> (84.9, -4)
  line L491 (84.9, -4) -> (84.9, -45.6)
  line L492 (84.9, -45.6) -> (4, -45.6)
  line L493 (4, -45.6) -> (4, -4)
  circle A0 centre (82.1501, -7.3501) radius 6
  circle A1 centre (7.147, -7.3545) radius 6
  circle A2 centre (7.1569, -38.2512) radius 6
  circle A3 centre (82.1501, -38.2512) radius 6
  line L494 (77.6535, -46.7993) -> (79.1535, -49.3974)
  line L495 (79.1535, -49.3974) -> (82.1535, -49.3974)
  line L496 (82.1535, -49.3974) -> (83.6535, -46.7993)
  line L497 (83.6535, -46.7993) -> (82.1535, -44.2013)
  line L498 (82.1535, -44.2013) -> (79.1535, -44.2013)
  line L499 (79.1535, -44.2013) -> (77.6535, -46.7993)
  line L500 (5.6535, -15.2993) -> (4.1535, -12.7013)
  line L501 (4.1535, -12.7013) -> (1.1535, -12.7013)
  line L502 (1.1535, -12.7013) -> (-0.3465, -15.2993)
  line L503 (-0.3465, -15.2993) -> (1.1535, -17.8974)
  line L504 (1.1535, -17.8974) -> (4.1535, -17.8974)
  line L505 (4.1535, -17.8974) -> (5.6535, -15.2993)
  line L506 (-0.3465, -22.2993) -> (1.1535, -24.8974)
  line L507 (1.1535, -24.8974) -> (4.1535, -24.8974)
  line L508 (4.1535, -24.8974) -> (5.6535, -22.2993)
  line L509 (5.6535, -22.2993) -> (4.1535, -19.7013)
  line L510 (1.1535, -19.7013) -> (-0.3465, -22.2993)
  line L511 (4.1535, -19.7013) -> (1.1535, -19.7013)
  line L512 (-0.3465, -29.2993) -> (1.1535, -31.8974)
  line L513 (1.1535, -31.8974) -> (4.1535, -31.8974)
  line L514 (4.1535, -31.8974) -> (5.6535, -29.2993)
  line L515 (5.6535, -29.2993) -> (4.1535, -26.7013)
  line L516 (1.1535, -26.7013) -> (-0.3465, -29.2993)
  line L517 (4.1535, -26.7013) -> (1.1535, -26.7013)
  line L518 (-0.3465, -36.2993) -> (1.1535, -38.8974)
  line L519 (1.1535, -38.8974) -> (4.1535, -38.8974)
  line L520 (4.1535, -38.8974) -> (5.6535, -36.2993)
  line L521 (5.6535, -36.2993) -> (4.1535, -33.7013)
  line L522 (1.1535, -33.7013) -> (-0.3465, -36.2993)
  line L523 (4.1535, -33.7013) -> (1.1535, -33.7013)
  line L524 (83.6535, -15.2993) -> (85.1535, -17.8974)
  line L525 (85.1535, -17.8974) -> (88.1535, -17.8974)
  line L526 (88.1535, -17.8974) -> (89.6535, -15.2993)
  line L527 (89.6535, -15.2993) -> (88.1535, -12.7013)
  line L528 (88.1535, -12.7013) -> (85.1535, -12.7013)
  line L529 (85.1535, -12.7013) -> (83.6535, -15.2993)
  line L530 (83.6535, -22.2993) -> (85.1535, -24.8974)
  line L531 (85.1535, -24.8974) -> (88.1535, -24.8974)
  line L532 (88.1535, -24.8974) -> (89.6535, -22.2993)
  line L533 (89.6535, -22.2993) -> (88.1535, -19.7013)
  line L534 (85.1535, -19.7013) -> (83.6535, -22.2993)
  line L535 (88.1535, -19.7013) -> (85.1535, -19.7013)
  line L536 (83.6535, -29.2993) -> (85.1535, -31.8974)
  line L537 (85.1535, -31.8974) -> (88.1535, -31.8974)
  line L538 (88.1535, -31.8974) -> (89.6535, -29.2993)
  line L539 (89.6535, -29.2993) -> (88.1535, -26.7013)
  line L540 (85.1535, -26.7013) -> (83.6535, -29.2993)
  line L541 (88.1535, -26.7013) -> (85.1535, -26.7013)
  line L542 (83.6535, -43.2993) -> (85.1535, -45.8974)
  line L543 (85.1535, -45.8974) -> (88.1535, -45.8974)
  line L544 (88.1535, -45.8974) -> (89.6535, -43.2993)
  line L545 (89.6535, -43.2993) -> (88.1535, -40.7013)
  line L546 (85.1535, -40.7013) -> (83.6535, -43.2993)
  line L547 (88.1535, -40.7013) -> (85.1535, -40.7013)
  line L548 (77.6535, -4.7993) -> (79.1535, -7.3974)
  line L549 (79.1535, -7.3974) -> (82.1535, -7.3974)
  line L550 (82.1535, -7.3974) -> (83.6535, -4.7993)
  line L551 (83.6535, -4.7993) -> (82.1535, -2.2013)
  line L552 (82.1535, -2.2013) -> (79.1535, -2.2013)
  line L553 (79.1535, -2.2013) -> (77.6535, -4.7993)
  line L554 (-0.3465, -43.2993) -> (1.1535, -45.8974)
  line L555 (1.1535, -45.8974) -> (4.1535, -45.8974)
  line L556 (4.1535, -45.8974) -> (5.6535, -43.2993)
  line L557 (5.6535, -43.2993) -> (4.1535, -40.7013)
  line L558 (4.1535, -40.7013) -> (1.1535, -40.7013)
  line L559 (1.1535, -40.7013) -> (-0.3465, -43.2993)
  circle A4 centre (13.147, -31.3523) radius 4
  circle A5 centre (13.147, -31.3523) radius 2
  circle A6 centre (13.147, -7.3523) radius 2
  circle A7 centre (13.147, -7.3523) radius 4
  line L560 (77.6535, -8.2993) -> (76.1535, -5.7013)
  line L561 (76.1535, -5.7013) -> (73.1535, -5.7013)
  line L562 (73.1535, -5.7013) -> (71.6535, -8.2993)
  line L563 (71.6535, -8.2993) -> (73.1535, -10.8974)
  line L564 (73.1535, -10.8974) -> (76.1535, -10.8974)
  line L565 (76.1535, -10.8974) -> (77.6535, -8.2993)
  line L566 (71.6535, -8.2993) -> (73.1535, -10.8974)
  line L567 (73.1535, -10.8974) -> (76.1535, -10.8974)
  line L568 (76.1535, -10.8974) -> (77.6535, -8.2993)
  line L569 (77.6535, -8.2993) -> (76.1535, -5.7013)
  line L570 (76.1535, -5.7013) -> (73.1535, -5.7013)
  line L571 (73.1535, -5.7013) -> (71.6535, -8.2993)
  circle A8 centre (37.147, -7.3523) radius 4.25
  point P0 (44.6535, -25.7993)
  point P1 (44.6535, -25.7993)
  point P2 (44.6535, -25.7993)
  point P3 (86.9, -47.6)
  point P4 (82.1501, -7.3501)
  point P5 (7.147, -7.3545)
  point P6 (7.1569, -38.2512)
  point P7 (82.1501, -38.2512)
  point P8 (0, -43.2993)
  point P9 (88.9, -43.2993)
  point P10 (74.6535, -43.2993)
  point P11 (50.6535, -43.2993)
  point P12 (38.6535, -43.2993)
  point P13 (14.6535, -43.2993)
  point P14 (14.6535, -43.2993)
  dimension "d87" = 12
  dimension "d88" = 12
  dimension "d89" = 12
  dimension "d90" = 12
  dimension "d138" = 4
  dimension "d139" = 8
  dimension "d140" = 4
  dimension "d141" = 8
  dimension "d237" = 8.5
  measures "d87" diameter of A0
  measures "d88" diameter of A1
  measures "d89" diameter of A2
  measures "d90" diameter of A3
  measures "d138" diameter of A5
  measures "d139" diameter of A4
  measures "d140" diameter of A6
  measures "d141" diameter of A7
  measures "d237" diameter of A8
extrude "Extrude7" cut sketch "Bottom Honeycomb" along normal blind 2 contours L4 L5 L6 L7 L8 L9 | L10 L11 L12 L13 L14 L15 | L16 L17 L18 L19 L20 L21 | L22 L23 L24 L25 L26 L27 | L28 L29 L30 L31 L32 L33 | L34 L35 L36 L37 L38 L39 | L40 L41 L42 L43 L44 L45 | L46 L47 L48 L49 L50 L51 | L52 L53 L54 L55 L56 L57 | L58 L59 L62 L63 A4 | L59 L60 L61 L62 A4 A5 | L60 L61 A5 | L256 L257 L258 A2 A4 | L256 L259 L260 L261 A2 A4 | L258 A2 A4 | L258 L259 A2 A4 | L322 L323 L325 L326 A1 A6 A7 | L325 A1 A6 | L322 L326 L327 A7 | L324 L325 A1 A6 | L323 L324 A1 A6 | L352 L353 L354 L355 L356 L357 A0 L560 L561 L562 L563 L564 L565 L566 L567 L568 L569 L570 L571 | L352 L356 A0 L560 L565 L568 L569 | L166 L167 L168 L169 L170 L171 A8 | L166 L167 A8 | L334 L335 L336 L337 L339 A8 | L334 L338 L339 A8 | L286 L287 L288 L289 L290 L291 A3 | L286 L290 A3 | L64 L65 L66 L67 L68 L69 | L70 L71 L72 L73 L74 L75 | L76 L77 L78 L79 L80 L81 | L82 L83 L84 L85 L86 L87 | L88 L89 L90 L91 L92 L93 | L94 L95 L96 L97 L98 L99 | L100 L101 L102 L103 L104 L105 | L106 L107 L108 L109 L110 L111 | L112 L113 L114 L115 L116 L117 | L118 L119 L120 L121 L122 L123 | L124 L125 L126 L127 L128 L129 | L130 L131 L132 L133 L134 L135 | L136 L137 L138 L139 L140 L141 | L142 L143 L144 L145 L146 L147 | L148 L149 L150 L151 L152 L153 | L154 L155 L156 L157 L158 L159 | L160 L161 L162 L163 L164 L165 | L172 L173 L174 L175 L176 L177 | L178 L179 L180 L181 L182 L183 | L184 L185 L186 L187 L188 L189 | L190 L191 L192 L193 L194 L195 | L196 L197 L198 L199 L200 L201 | L202 L203 L204 L205 L206 L207 | L208 L209 L210 L211 L212 L213 | L214 L215 L216 L217 L218 L219 | L220 L221 L222 L223 L224 L225 | L226 L227 L228 L229 L230 L231 | L232 L233 L234 L235 L236 L237 | L238 L239 L240 L241 L242 L243 | L244 L245 L246 L247 L248 L249 | L250 L251 L252 L253 L254 L255 | L262 L263 L264 L265 L266 L267 | L268 L269 L270 L271 L272 L273 | L274 L275 L276 L277 L278 L279 | L280 L281 L282 L283 L284 L285 | L292 L293 L294 L295 L296 L297 | L298 L299 L300 L301 L302 L303 | L304 L305 L306 L307 L308 L309 | L310 L311 L312 L313 L314 L315 | L316 L317 L318 L319 L320 L321 | L328 L329 L330 L331 L332 L333 | L340 L341 L342 L343 L344 L345 | L346 L347 L348 L349 L350 L351 picked at (13.1638, -30.2044) picked at (12.5872, -8.3344) picked at (13.7393, -7.857) bodies 1
sketch "Fan Mount" plane through (0, 0, 0) normal (0, 1, 0) x (1, 0, 0)
  line L0 (13.147, -7.3523) -> (37.147, -7.3523) construction
  line L1 (37.147, -7.3523) -> (37.147, -31.3523) construction
  line L2 (37.147, -31.3523) -> (13.147, -31.3523) construction
  line L3 (13.147, -31.3523) -> (13.147, -7.3523) construction
  circle A0 centre (13.147, -31.3523) radius 1.5
  circle A1 centre (13.147, -31.3523) radius 4.25
  circle A2 centre (37.147, -31.3523) radius 4.25
  circle A3 centre (37.147, -31.3523) radius 1.5
  circle A4 centre (37.147, -7.3523) radius 1.5
  circle A5 centre (37.147, -7.3523) radius 4.25
  circle A6 centre (13.147, -7.3523) radius 1.5
  circle A7 centre (13.147, -7.3523) radius 4.25
  circle A8 centre (7.147, -7.3545) radius 3.25
  circle A9 centre (7.147, -7.3545) radius 3.25
  circle A10 centre (7.147, -7.3545) radius 3.25
  circle A11 centre (37.147, -7.3523) radius 4.25
  point P0 (7.147, -7.3545)
  dimension "d63" = 24
  dimension "d64" = 24
  dimension "d65" = 3
  dimension "d66" = 8.5
  dimension "d67" = 3
  dimension "d68" = 8.5
  dimension "d69" = 3
  dimension "d70" = 8.5
  dimension "d71" = 3
  dimension "d72" = 8.5
  measures "d63" distance of L0.start L0.end
  measures "d64" distance of L0.start L2.end
  measures "d65" diameter of A0
  measures "d66" diameter of A1
  measures "d67" diameter of A3
  measures "d68" diameter of A2
  measures "d69" diameter of A4
  measures "d70" diameter of A5
  measures "d71" diameter of A6
  measures "d72" diameter of A7